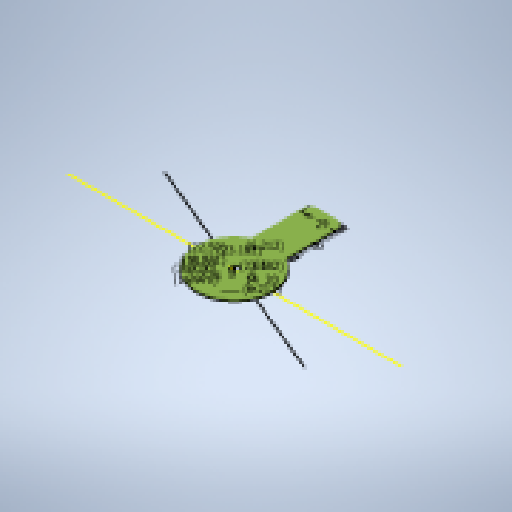
# Autodesk Inventor part: 038
Saved by Autodesk Inventor 2023 (Build 270158000, 158)
## iProperties
Created: 2022-04-25
Part Number: 038
Material: GFRC
Document SubType Name: Modeling
Designer: vmiguel
Density: 1.7 g/cm^3
Appearance: Olive Green
Author: vmiguel
Autodesk Inventor part; units mm, degrees
ref_plane "YZ Plane" through (0, 0, 0) normal (1, 0, 0) x (0, 1, 0)
ref_plane "XZ Plane" through (0, 0, 0) normal (0, 1, 0) x (-1, 0, 0)
ref_plane "XY Plane" through (0, 0, 0) normal (0, 0, 1) x (1, 0, 0)
sketch "Sketch1" plane through (0, 0, 0) normal (0, 1, 0) x (-1, 0, 0)
  circle A0 centre (0, 0) radius 32.5
  circle A1 centre (0, 0) radius 4
  line L0 (-14.5, -79.0861) -> (-14.5, -29.0861)
  line L1 (-14.5, -29.0861) -> (14.5, -29.0861) construction
  line L2 (14.5, -29.0861) -> (14.5, -79.0861)
  line L3 (14.5, -79.0861) -> (-14.5, -79.0861)
  line L4 (-14.5, -79.0861) -> (14.5, -29.0861) construction
  line L5 (-14.5, -29.0861) -> (14.5, -79.0861) construction
  line L6 (0, 0) -> (16.9706, 16.9706) construction
  circle A2 centre (16.9706, 16.9706) radius 1.6
  circle A3 centre (-23.1822, 6.2117) radius 1.6
  circle A4 centre (6.2117, -23.1822) radius 1.6
  circle A5 centre (0, 0) radius 10
  circle A6 centre (0, 0) radius 7
  line L7 (-7, 0) -> (-4.9497, 4.9497)
  line L8 (-4.9497, 4.9497) -> (0, 7)
  line L9 (0, 7) -> (4.9497, 4.9497)
  line L10 (4.9497, 4.9497) -> (7, 0)
  line L11 (7, 0) -> (4.9497, -4.9497)
  line L12 (4.9497, -4.9497) -> (0, -7)
  line L13 (0, -7) -> (-4.9497, -4.9497)
  line L14 (-4.9497, -4.9497) -> (-7, 0)
  line L15 (-101.397, 42) -> (101.397, -42)
  line L16 (-141.9558, 0) -> (141.9558, 0) projected
  point P0 (0, -54.0861)
  point P1 (0, -54.0861)
  point P2 (5.9749, -2.4749)
  point P3 (0, 0)
  dimension "d16" = 14
  dimension "d0" = 65
  dimension "d1" = 8
  dimension "d4" = 29
  dimension "d5" = 50
  dimension "d6" = 24
  dimension "d8" = 3.2
  dimension "d11" = 360
  dimension "d14" = 135
  dimension "d15" = 20
  dimension "d17" = 22.5
  dimension "d18" = 6.2117
  dimension "d19" = 23.1822
  dimension "d20" = 16.9706
  dimension "d21" = 16.9706
  dimension "d22" = 23.1822
  dimension "d23" = 6.2117
  constraints: 32 end point, 6 centre point, 6 coincident, 5 midpoint, 2 parallel, 2 point on circle, 2 vertical alignment, 1 perpendicular, 1 point on line, 29 other
  measures "d0" diameter of A0
  measures "d1" diameter of A1
  measures "d4" distance of L2.end L0.start
  measures "d5" distance of L0.start L0.end
  measures "d6" distance of L6.start L6.end
  measures "d8" diameter of A2
  measures "d14" angle of L2 L6
  measures "d15" diameter of A5
  measures "d17" angle of L16 L15
  measures "d18" horizontal distance of A4.centre point (0, 0)
  measures "d19" vertical distance of A4.centre point (0, 0)
  measures "d20" horizontal distance of L6.end point (0, 0)
  measures "d21" horizontal distance of A2.centre point (0, 0)
  measures "d22" horizontal distance of point (0, 0) A3.centre
  measures "d23" vertical distance of A3.centre point (0, 0)
extrude "Extrusion1" add sketch "Sketch1" along normal blind 1.6 contours A0 L16 A5 L15 | A0 L2 L3 L0 | A0 L15 A5 L16 | L15 A5 L16 A0 | A0 L16 A5 L15 | L16 A6 L15 A5 | A5 L15 A6 L16 | L15 A6 L16 A5 | A5 L16 A6 L15 | L14 A6 | A6 L15 L7 | L16 A1 L15 L11 L12 L13 L14 | L7 L15 A1 L16 | L15 L11 A6 | A6 L11 L15 | A6 L7 L15 | L13 A6 | L7 L8 L9 L10 L16 A1 L15 | L10 A6 | L11 L15 A1 L16 | A6 L12 | A6 L8 | L9 A6
fillet "Fillet1" radius 5 2 edges at (-14.5, 0.8, -79.0861) (14.5, 0.8, -79.0861)
body "Solid1"
